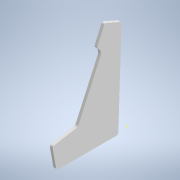
# Autodesk Inventor part: Arcade_Right
Saved by Autodesk Inventor 2022 (Build 260153000, 153)
## iProperties
Created: 2023-12-22
Part Number: Arcade_Right
Material: Generic
Document SubType Name: Modeling
Designer: Petr Černý
Density: 1 g/cm^3
Appearance: Default
Author: Petr Černý
Autodesk Inventor part; units mm, degrees
ref_plane "YZ Plane" through (0, 0, 0) normal (1, 0, 0) x (0, 1, 0)
ref_plane "XZ Plane" through (0, 0, 0) normal (0, 1, 0) x (-1, 0, 0)
ref_plane "XY Plane" through (0, 0, 0) normal (0, 0, 1) x (1, 0, 0)
sketch "Sketch1" plane through (0, 0, 0) normal (1, 0, 0) x (0, 1, 0)
  line L0 (9.8481, 428.814) -> (120.1519, 448.2635)
  line L1 (131.7365, 440.1519) -> (154.2135, 312.6787)
  line L2 (0, 78.3368) -> (0, 427.0775)
  line L3 (0, 417.0775) -> (0, 78.3368)
  line L4 (503.1119, 189.3047) -> (590.8645, 150.2346)
  line L5 (595.9326, 137.0318) -> (559.5861, 55.3964)
  line L6 (494.9423, 192.942) -> (494.9423, 192.942)
  line L7 (442.0149, 172.9748) -> (165.6696, 297.928)
  arc A0 (442.0149, 172.9748) -> (490.9347, 186.0198) centre (458.495, 209.4221) ccw
  arc A1 (154.2135, 312.6787) -> (165.6696, 297.928) centre (173.9096, 316.1516) ccw
  arc A2 (131.7365, 440.1519) -> (120.1519, 448.2635) centre (121.8884, 438.4154) ccw
  line L8 (9.8481, 428.814) -> (0, 417.0775)
  arc A3 (595.9326, 137.0318) -> (590.8645, 150.2346) centre (586.7972, 141.0991) ccw
  arc A4 (503.1119, 189.3047) -> (490.9347, 186.0198) centre (499.0446, 180.1692) ccw
  line L9 (9.651, 68.3429) -> (550.1017, 49.4699)
  arc A5 (550.1017, 49.4699) -> (559.5861, 55.3964) centre (550.4507, 59.4638) ccw
  arc A6 (0, 78.3368) -> (9.651, 68.3429) centre (10, 78.3368) ccw
  point P0 (0, 0)
  point P1 (0, 0)
  point P2 (130, 450)
  point P3 (156.0472, 302.2788)
  point P4 (0, 0)
  point P5 (534.922, 0)
  point P6 (600, 146.1672)
  point P7 (478.4622, 156.4947)
  point P8 (0, 427.0775)
  point P9 (537.6655, 6.1619)
  point P10 (0, 417.0775)
  dimension "d0" = 130
  dimension "d1" = 404.922
  dimension "d3" = 150
  dimension "d5" = 115
  dimension "d7" = 10
  dimension "d9" = 40
  dimension "d10" = 40
  dimension "d11" = 20
  dimension "d12" = 10
  dimension "d13" = 10
  dimension "d14" = 10
  dimension "d21" = 10
  constraints: 20 end point, 15 point on circle, 15 point on line, 14 tangent, 7 centre point, 3 perpendicular, 1 equal radius
  measures "d0" distance from line of point (130, 450) L2
  measures "d1" horizontal distance of point (130, 450) point (534.922, 0)
  measures "d3" distance of point (130, 450) point (156.047, 302.279)
  measures "d5" distance of L6.start point (600, 146.167)
  measures "d7" angle of L1 L3
  measures "d9" distance of L6.start point (478.462, 156.495)
  measures "d10" radius of A0
  measures "d11" radius of A1
  measures "d12" radius of A2
  measures "d13" distance of L8.start point (0, 427.077)
  measures "d14" distance of L8.end point (0, 427.077)
  measures "d21" radius of A5
extrude "Extrusion1" add sketch "Sketch1" along normal blind 16
sketch "Sketch2" plane through (0, 0, 0) normal (-1, 0, 0) x (0, 0, 1)
  point P0 (0, 0)
sketch "Sketch3" plane through (0, 0, 0) normal (-1, 0, 0) x (0, 0, 1)
  line L0 (171.0338, 494.9772) -> (173.8576, 488.6347) projected
  line L1 (166.9664, 504.1126) -> (130.324, 487.7983) projected
  line L2 (130.324, 487.7983) -> (274.7158, 163.4898) projected
  line L3 (274.7158, 163.4898) -> (219.9031, 139.0856) projected
  line L4 (219.9031, 139.0856) -> (223.9704, 129.9501) projected
  line L5 (223.9704, 129.9501) -> (278.7831, 154.3544) projected
  line L6 (278.7831, 154.3544) -> (288.9516, 131.5158) projected
  line L7 (288.9516, 131.5158) -> (298.087, 135.5831) projected
  line L8 (298.087, 135.5831) -> (143.5268, 482.7303) projected
  line L9 (143.5268, 482.7303) -> (171.0338, 494.9772) projected
  line L10 (173.8576, 488.6347) -> (182.9931, 492.702) projected
  line L11 (182.9931, 492.702) -> (141.0991, 586.7972) projected
  line L12 (141.0991, 586.7972) -> (131.9637, 582.7298) projected
  line L13 (301.7603, 135.8301) -> (426.8309, 113.7768) projected
  line L14 (426.8309, 113.7768) -> (407.5559, 4.4631) projected
  line L15 (407.5559, 4.4631) -> (417.404, 2.7267) projected
  line L16 (417.404, 2.7267) -> (438.4154, 121.8884) projected
  line L17 (438.4154, 121.8884) -> (303.4968, 145.6782) projected
  line L18 (303.4968, 145.6782) -> (301.7603, 135.8301) projected
  line L19 (428.814, 9.8481) -> (417.0775, 0) projected
  line L20 (417.0775, 0) -> (78.3368, 0) projected
  line L21 (55.3964, 559.5861) -> (137.0318, 595.9326) projected
  arc A0 (150.2346, 590.8645) -> (137.0318, 595.9326) centre (141.0991, 586.7972) ccw projected
  line L22 (150.2346, 590.8645) -> (189.3047, 503.1119) projected
  arc A1 (186.0198, 490.9347) -> (189.3047, 503.1119) centre (180.1692, 499.0446) ccw projected
  arc A2 (186.0198, 490.9347) -> (172.9748, 442.0149) centre (209.4221, 458.495) ccw projected
  line L23 (172.9748, 442.0149) -> (297.928, 165.6696) projected
  arc A3 (297.928, 165.6696) -> (312.6787, 154.2135) centre (316.1516, 173.9096) ccw projected
  line L24 (312.6787, 154.2135) -> (440.1519, 131.7365) projected
  arc A4 (448.2635, 120.1519) -> (440.1519, 131.7365) centre (438.4154, 121.8884) ccw projected
  line L25 (448.2635, 120.1519) -> (428.814, 9.8481) projected
  line L26 (171.0338, 494.9772) -> (173.8576, 488.6347) projected
  line L27 (166.9664, 504.1126) -> (130.324, 487.7983) projected
  line L28 (130.324, 487.7983) -> (274.7158, 163.4898) projected
  line L29 (274.7158, 163.4898) -> (219.9031, 139.0856) projected
  line L30 (219.9031, 139.0856) -> (223.9704, 129.9501) projected
  line L31 (223.9704, 129.9501) -> (278.7831, 154.3544) projected
  line L32 (278.7831, 154.3544) -> (288.9516, 131.5158) projected
  line L33 (288.9516, 131.5158) -> (298.087, 135.5831) projected
  line L34 (298.087, 135.5831) -> (143.5268, 482.7303) projected
  line L35 (143.5268, 482.7303) -> (171.0338, 494.9772) projected
  line L36 (173.8576, 488.6347) -> (182.9931, 492.702) projected
  line L37 (182.9931, 492.702) -> (141.0991, 586.7972) projected
  line L38 (141.0991, 586.7972) -> (131.9637, 582.7298) projected
  line L39 (301.7603, 135.8301) -> (426.8309, 113.7768) projected
  line L40 (426.8309, 113.7768) -> (407.5559, 4.4631) projected
  line L41 (407.5559, 4.4631) -> (417.404, 2.7267) projected
  line L42 (417.404, 2.7267) -> (438.4154, 121.8884) projected
  line L43 (438.4154, 121.8884) -> (303.4968, 145.6782) projected
  line L44 (303.4968, 145.6782) -> (301.7603, 135.8301) projected
  line L45 (428.814, 9.8481) -> (417.0775, 0) projected
  line L46 (417.0775, 0) -> (78.3368, 0) projected
  line L47 (55.3964, 559.5861) -> (137.0318, 595.9326) projected
  arc A5 (150.2346, 590.8645) -> (137.0318, 595.9326) centre (141.0991, 586.7972) ccw projected
  line L48 (150.2346, 590.8645) -> (189.3047, 503.1119) projected
  arc A6 (186.0198, 490.9347) -> (189.3047, 503.1119) centre (180.1692, 499.0446) ccw projected
  arc A7 (186.0198, 490.9347) -> (172.9748, 442.0149) centre (209.4221, 458.495) ccw projected
  line L49 (172.9748, 442.0149) -> (297.928, 165.6696) projected
  arc A8 (297.928, 165.6696) -> (312.6787, 154.2135) centre (316.1516, 173.9096) ccw projected
  line L50 (312.6787, 154.2135) -> (440.1519, 131.7365) projected
  arc A9 (448.2635, 120.1519) -> (440.1519, 131.7365) centre (438.4154, 121.8884) ccw projected
  line L51 (448.2635, 120.1519) -> (428.814, 9.8481) projected
  line L52 (417.404, 2.7267) -> (438.4154, 121.8884) projected
  line L53 (58.3797, 539.0217) -> (136.0311, 573.5943)
  line L54 (54.3124, 548.1571) -> (141.0991, 586.7972)
  line L55 (136.0311, 573.5943) -> (131.9637, 582.7298)
  line L56 (141.0991, 586.7972) -> (182.9931, 492.702)
  line L57 (182.9931, 492.702) -> (173.8576, 488.6347)
  line L58 (166.9664, 504.1126) -> (136.0311, 573.5943)
  line L59 (166.9664, 504.1126) -> (130.324, 487.7983)
  line L60 (130.324, 487.7983) -> (274.7158, 163.4898)
  line L61 (274.7158, 163.4898) -> (219.9031, 139.0856)
  line L62 (219.9031, 139.0856) -> (223.9704, 129.9501)
  line L63 (223.9704, 129.9501) -> (278.7831, 154.3544)
  line L64 (278.7831, 154.3544) -> (288.9516, 131.5158)
  line L65 (288.9516, 131.5158) -> (298.087, 135.5831)
  line L66 (298.087, 135.5831) -> (143.5268, 482.7303)
  line L67 (143.5268, 482.7303) -> (171.0338, 494.9772)
  line L68 (171.0338, 494.9772) -> (173.8576, 488.6347)
  line L69 (303.4968, 145.6782) -> (301.7603, 135.8301)
  line L70 (301.7603, 135.8301) -> (426.8309, 113.7768)
  line L71 (426.8309, 113.7768) -> (407.5559, 4.4631)
  line L72 (407.5559, 4.4631) -> (417.404, 2.7267)
  line L73 (417.404, 2.7267) -> (438.4154, 121.8884)
  line L74 (438.4154, 121.8884) -> (303.4968, 145.6782)
  line L75 (131.9637, 582.7298) -> (54.3123, 548.1572) projected
  line L76 (54.3123, 548.1572) -> (58.3797, 539.0217) projected
  line L77 (58.3797, 539.0217) -> (136.0311, 573.5943) projected
  line L78 (136.0311, 573.5943) -> (166.9664, 504.1126) projected
  line L79 (68.3429, 9.651) -> (49.4699, 550.1017) projected
  arc A10 (55.3964, 559.5861) -> (49.4699, 550.1017) centre (59.4638, 550.4507) ccw projected
  arc A11 (68.3429, 9.651) -> (78.3368, 0) centre (78.3368, 10) ccw projected
  line L80 (131.9637, 582.7298) -> (54.3123, 548.1572) projected
  line L81 (54.3123, 548.1572) -> (58.3797, 539.0217) projected
  line L82 (58.3797, 539.0217) -> (136.0311, 573.5943) projected
  line L83 (136.0311, 573.5943) -> (166.9664, 504.1126) projected
  line L84 (68.3429, 9.651) -> (49.4699, 550.1017) projected
  arc A12 (55.3964, 559.5861) -> (49.4699, 550.1017) centre (59.4638, 550.4507) ccw projected
  arc A13 (68.3429, 9.651) -> (78.3368, 0) centre (78.3368, 10) ccw projected
  line L85 (54.3123, 548.1572) -> (58.3797, 539.0217)
  line L86 (73.2484, 352.9229) -> (142.3938, 197.6203) projected
  line L87 (142.3938, 197.6203) -> (156.0969, 203.7213) projected
  line L88 (156.0969, 203.7213) -> (86.9516, 359.024) projected
  line L89 (86.9516, 359.024) -> (73.2484, 352.9229) projected
  line L90 (73.2484, 352.9229) -> (142.3938, 197.6203) projected
  line L91 (142.3938, 197.6203) -> (156.0969, 203.7213) projected
  line L92 (156.0969, 203.7213) -> (86.9516, 359.024) projected
  line L93 (86.9516, 359.024) -> (73.2484, 352.9229) projected
  line L94 (86.9516, 359.024) -> (156.0969, 203.7213)
  line L95 (142.3938, 197.6203) -> (156.0969, 203.7213)
  line L96 (142.3938, 197.6203) -> (73.2484, 352.9229)
  line L97 (73.2484, 352.9229) -> (86.9516, 359.024)
  point P0 (0, 0)
  point P1 (131.9642, 582.73)
  constraints: 54 end point, 15 perpendicular, 6 collinear, 3 point on line, 1 parallel
extrude "Extrusion2" cut sketch "Sketch3" against normal blind 7 contours L9 L8 L7 L6 L5 L4 L3 L2 L1 L58 L55 L12 L11 L10 L0 | L55 L53 L76 L54 | L18 L17 L16 L15 L14 L13 | L89 L88 L87 L86
equation "\"d14\" = d13"
body "Solid1"
